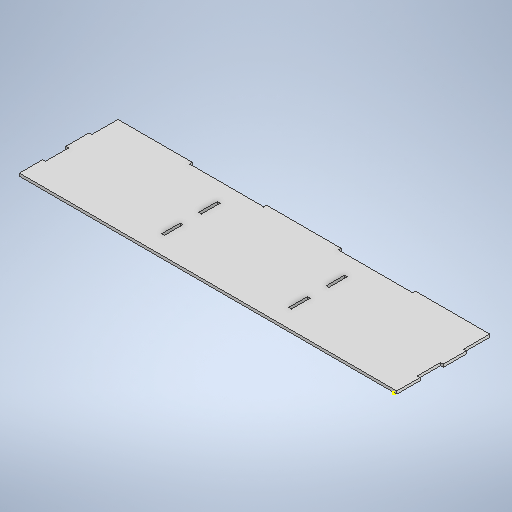
# Autodesk Inventor part: Base sup e inf
Saved by Autodesk Inventor 2025.1 (Build 291241020, 241B)
## iProperties
Created: 2024-11-13
Part Number: Base sup e inf
Material: Generic
Document SubType Name: Modeling
Designer: marco
Density: 1 g/cm^3
Appearance: Default
Author: marco
Autodesk Inventor part; units mm, degrees
ref_plane "YZ Plane" through (0, 0, 0) normal (1, 0, 0) x (0, 1, 0)
ref_plane "XZ Plane" through (0, 0, 0) normal (0, 1, 0) x (-1, 0, 0)
ref_plane "XY Plane" through (0, 0, 0) normal (0, 0, 1) x (1, 0, 0)
sketch "Sketch1" plane through (0, 0, 0) normal (0, 1, 0) x (-1, 0, 0)
  line L0 (0, 0) -> (400, 0)
  line L1 (400, 0) -> (400, -100)
  line L2 (400, -100) -> (0, -100)
  line L3 (0, -100) -> (0, 0)
  line L4 (400, -100) -> (400, -103)
  line L5 (400, -103) -> (320, -103)
  line L6 (320, -103) -> (320, -100)
  line L7 (0, -100) -> (0, -103)
  line L8 (0, -103) -> (80, -103)
  line L9 (80, -103) -> (80, -100)
  line L10 (240, -100) -> (240, -103)
  line L11 (240, -103) -> (160, -103)
  line L12 (160, -103) -> (160, -100)
  line L13 (400, 0) -> (403, 0)
  line L14 (403, 0) -> (403, -25)
  line L15 (403, -25) -> (400, -25)
  line L16 (400, -25) -> (400, -50)
  line L17 (400, -50) -> (403, -50)
  line L18 (403, -50) -> (403, -75)
  line L19 (403, -75) -> (400, -75)
  line L20 (200, 0) -> (200, -100) construction
  line L21 (0, 0) -> (0, -100)
  line L22 (0, 0) -> (-3, 0)
  line L23 (-3, 0) -> (-3, -25)
  line L24 (-3, -25) -> (0, -25)
  line L25 (0, -25) -> (0, -50)
  line L26 (0, -50) -> (-3, -50)
  line L27 (-3, -50) -> (-3, -75)
  line L28 (-3, -75) -> (0, -75)
  line L29 (0, 0) -> (130, 0)
  line L30 (130, 0) -> (264, 0)
  line L31 (130, 0) -> (133, 0)
  line L32 (133, 0) -> (267, 0)
  line L33 (267, 0) -> (270, 0)
  line L34 (130, -20) -> (133, -20)
  line L35 (130, -20) -> (130, -40)
  line L36 (130, -40) -> (133, -40)
  line L37 (130, -80) -> (133, -80)
  line L38 (130, -80) -> (130, -60)
  line L39 (130, -60) -> (133, -60)
  line L40 (133, -20) -> (133, -40)
  line L41 (133, -60) -> (133, -80)
  line L42 (270, -20) -> (267, -20)
  line L43 (270, -20) -> (270, -40)
  line L44 (270, -40) -> (267, -40)
  line L45 (270, -80) -> (267, -80)
  line L46 (270, -80) -> (270, -60)
  line L47 (270, -60) -> (267, -60)
  line L48 (267, -20) -> (267, -40)
  line L49 (267, -60) -> (267, -80)
  dimension "d0" = 400
  dimension "d1" = 100
  dimension "d2" = 3
  dimension "d3" = 80
  dimension "d4" = 3
  dimension "d5" = 80
  dimension "d7" = 3
  dimension "d8" = 80
  dimension "d9" = 3
  dimension "d10" = 25
  dimension "d11" = 25
  dimension "d12" = 3
  dimension "d13" = 25
  dimension "d16" = 130
  dimension "d17" = 134
  dimension "d18" = 3
  dimension "d19" = 134
  dimension "d20" = 3
  dimension "d21" = 20
  dimension "d22" = 20
  dimension "d24" = 20
  constraints: 100 end point, 21 point on line, 15 symmetric about line, 8 perpendicular, 4 midpoint, 3 equal length, 2 horizontal, 2 vertical
  measures "d0" distance of L1.end L2.end
  measures "d1" distance of L0.end L1.end
  measures "d2" distance of L1.end L4.end
  measures "d3" distance of L4.end L5.end
  measures "d4" distance of L2.end L7.end
  measures "d5" distance of L7.end L8.end
  measures "d7" distance of L10.start L10.end
  measures "d8" distance of L10.end L11.end
  measures "d9" distance of L0.end L13.end
  measures "d10" distance of L13.end L14.end
  measures "d11" distance of L15.end L16.end
  measures "d12" distance of L16.end L17.end
  measures "d13" distance of L17.end L18.end
  measures "d16" distance of L0.start L29.end
  measures "d17" distance of L29.end L30.end
  measures "d18" distance of L29.end L31.end
  measures "d19" distance of L31.end L32.end
  measures "d20" distance of L32.end L33.end
  measures "d21" distance of L29.end L34.start
  measures "d22" distance of L34.start L35.end
  measures "d24" distance of L37.start L38.end
extrude "Extrusion1" add sketch "Sketch1" along normal blind 3
sketch "Sketch2" plane through (0, 0, 0) normal (0, -1, 0) x (1, 0, 0)
  point P0 (0, 0)
  point P1 (-394.1596, -5.7675)
  constraints: 1 other
body "Solid1"
